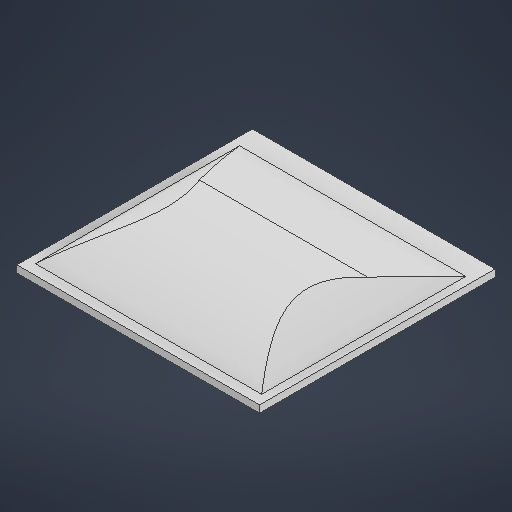
# Autodesk Inventor part: Obudowa
Saved by Autodesk Inventor 2026 (Build 300175000, 175)
## iProperties
Created: 2025-04-26
Part Number: Obudowa
Material: Generic
Document SubType Name: Modeling
Designer: isan
Density: 1 g/cm^3
Appearance: Default
Author: isan
Autodesk Inventor part; units mm, degrees
ref_plane "YZ Plane" through (0, 0, 0) normal (1, 0, 0) x (0, 1, 0)
ref_plane "XZ Plane" through (0, 0, 0) normal (0, 1, 0) x (-1, 0, 0)
ref_plane "XY Plane" through (0, 0, 0) normal (0, 0, 1) x (1, 0, 0)
sketch "Sketch1" plane through (0, 0, 0) normal (0, 0, 1) x (1, 0, 0)
  line L0 (-34, -33) -> (34, -33)
  line L1 (34, -33) -> (34, 33)
  line L2 (34, 33) -> (-34, 33)
  line L3 (-34, 33) -> (-34, -33)
  line L4 (-34, -33) -> (34, 33) construction
  line L5 (34, -33) -> (-34, 33) construction
  point P0 (0, 0)
  dimension "d0" = 68
  dimension "d1" = 66
  constraints: 12 end point, 2 midpoint, 2 parallel, 1 horizontal, 1 perpendicular
  measures "d0" distance of L1.end L2.end
  measures "d1" distance of L0.end L1.end
extrude "Extrusion1" add sketch "Sketch1" along normal blind 2
sketch "Sketch2" plane through (-34, -33, 0) normal (-1, 0, 0) x (0, 0, 1)
  line L0 (0, 0) -> (0, 66) construction
  line L1 (0, 66) -> (0, 0)
  line L2 (0, 65.9635) -> (0, 0)
  arc A0 (7.4259, 40.744) -> (0, 65.9635) centre (-222.7937, -13.3415) ccw
  arc A1 (0, 0) -> (7.4259, 40.744) centre (-36.728, 27.7427) ccw
  point P0 (0, 33)
  constraints: 4 end point, 4 point on circle, 2 centre point, 2 collinear, 1 point on line
extrude "Extrusion2" add sketch "Sketch2" against normal blind 68
sketch "Sketch3" plane through (-34, 33, 0) normal (0, 1, 0) x (1, 0, 0)
  line L0 (0, 0) -> (68, 0) projected
  line L1 (0, -10.0891) -> (68, -10.0891) projected
  line L2 (68, 0) -> (0, 0)
  line L3 (0, -2) -> (68, -2) projected
  line L4 (68, -2) -> (0, -2)
  line L5 (0, -2) -> (0, 0)
  line L6 (0, 0) -> (68, 0)
  line L7 (68, 0) -> (68, -2)
  arc A0 (0, 0) -> (68, 0) centre (34, 36.5643) ccw
  point P0 (34, 0)
  point P1 (51.788, -10.0891)
  point P2 (65.7135, -2)
  point P3 (2.2865, -2)
  point P4 (16.212, -10.0891)
  constraints: 10 end point, 3 equal length, 2 point on circle, 1 centre point, 1 horizontal, 1 perpendicular
extrude "Extrusion3" cut sketch "Sketch3" against normal blind 68 contours A0 L3 L5 | L0 A0 L3 | L7 L3 A0 | L3 A0 L1 keep common part
body "Solid1"
